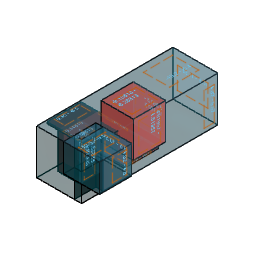
map kibo v7 (Autodesk Fusion 360 design; units mm, degrees)
Autodesk Fusion 360 part; units mm, degrees
sketch "Sketch1" plane through (0, 0, 0) normal (0, 0, 1) x (1, 0, 0)
  line L0 (12.5, 3.3758) -> (25, 3.3758)
  line L1 (25, 3.3758) -> (25, 41.3758)
  line L2 (25, 41.3758) -> (12.5, 41.3758)
  line L3 (12.5, 41.3758) -> (12.5, 3.3758)
  line L4 (93, 105.3758) -> (128, 105.3758)
  line L5 (128, 105.3758) -> (128, -41.5514)
  line L6 (23, 0.3758) -> (33, 0.3758)
  line L7 (33, 0.3758) -> (33, 9.3758)
  line L8 (33, 9.3758) -> (23, 9.3758)
  line L9 (23, 9.3758) -> (23, 0.3758)
  line L10 (20.327, 13.4945) -> (29.327, 13.4945)
  line L11 (29.327, 13.4945) -> (29.327, 22.4945)
  line L12 (29.327, 22.4945) -> (20.327, 22.4945)
  line L13 (20.327, 22.4945) -> (20.327, 13.4945)
  dimension "d1" = 12.5
  dimension "d2" = 38
  dimension "d4" = 102
  dimension "d5" = 103
  dimension "d12" = 10
  dimension "d13" = 9
  dimension "d15" = 10.5
  dimension "d17" = 3
  dimension "d50" = 9
  dimension "d51" = 9
  dimension "d53" = 3.673
  dimension "d54" = 13.1187
  constraint horizontal L0
  constraint vertical L1
  constraint horizontal L2
  constraint vertical L3
  constraint horizontal L4
  constraint perpendicular L4 L5
  constraint horizontal L6
  constraint vertical L7
  constraint horizontal L8
  constraint vertical L9
  constraint horizontal L10
  constraint vertical L11
  constraint horizontal L12
  constraint vertical L13
  measures "d1" distance of L1.end L2.end
  measures "d2" distance of L0.end L1.end
  measures "d4" distance of L0 L4
  measures "d5" distance of L1 L5
  measures "d12" distance of L6.start L6.end
  measures "d13" distance of L6.end L7.end
  measures "d15" distance of L3 L9
  measures "d17" distance of L0 L6
  measures "d50" distance of L10.start L12.end
  measures "d51" distance of L10.start L10.end
  measures "d53" distance of L7 L11
  measures "d54" distance of L6 L10
extrude "Extrude20" add sketch "Sketch1" against normal blind 48.1957 contours L1 L10 L11 L12 | L1 L10 L12 L13 makes body 1
extrude "Extrude17" add sketch "Sketch1" against normal blind 48 separate body contours L0 L1 L8 L9 makes body 2
extrude "Extrude15" add sketch "Sketch1" against normal blind 48 separate body contours L0 L1 L6 L7 L8 L9 makes body 3
extrude "Extrude12" add sketch "Sketch1" against normal blind 55.7 separate body contours L0 L1 L8 L9 makes body 4
extrude "Extrude5" add sketch "Sketch1" along normal blind 48 separate body contours L0 L1 L8 L9 makes body 5
extrude "Extrude4" add sketch "Sketch1" along normal blind 48 separate body contours L0 L1 L6 L7 L8 L9 makes body 6
extrude "Extrude2" add sketch "Sketch1" along normal blind 55.7 separate body contours L0 L1 L2 L3 L8 L9 L10 L12 L13 | L0 L1 L8 L9 | L1 L10 L12 L13 makes body 7
extrude "Extrude1" add sketch "Sketch1" along normal blind 12.5 separate body contours L0 L1 L2 L3 L8 L9 L10 L12 L13 | L0 L1 L8 L9 | L1 L10 L12 L13 makes body 8
extrude "Extrude3" cut sketch "Sketch1" along normal blind 43.2 contours L0 L1 L2 L3 L8 L9 L10 L12 L13 | L0 L1 L8 L9 | L1 L10 L12 L13 bodies 7 8
extrude "Extrude6" cut sketch "Sketch1" along normal blind 40.2 contours L0 L1 L6 L7 L8 L9 bodies 6
extrude "Extrude7" cut sketch "Sketch1" along normal blind 40.2 contours L0 L1 L8 L9 bodies 5
extrude "Extrude8" cut 1 faces at (20.8333, 16.0424, 55.7) along direction (0, 0, -1) blind 15 on bodies 7 bodies 5 7
extrude "Extrude9" cut 1 faces at (30.3333, 4.3758, 48) along direction (0, 0, -1) blind 10 on bodies 6 bodies 6
extrude "Extrude10" cut 1 faces at (23.6667, 7.3758, 40.7) along direction (0, 0, -1) blind 1 on bodies 5 bodies 5
extrude "Extrude11" add sketch "Sketch1" against normal blind 55.7 contours L0 L1 L2 L3 L8 L9 L10 L12 L13 | L1 L10 L12 L13 bodies 5 6 7 8
extrude "Extrude13" cut sketch "Sketch1" against normal blind 43.2 contours L0 L1 L2 L3 L8 L9 L10 L12 L13 | L1 L10 L12 L13 bodies 5
extrude "Extrude14" cut sketch "Sketch1" against normal blind 43.2 contours L0 L1 L8 L9 bodies 4
extrude "Extrude16" cut sketch "Sketch1" against normal blind 48 contours L0 L1 L8 L9 bodies 4
extrude "Extrude18" cut sketch "Sketch1" against normal blind 40.2 contours L0 L1 L6 L7 L8 L9 bodies 3
extrude "Extrude19" cut sketch "Sketch1" against normal blind 40.2 contours L0 L1 L8 L9 bodies 2
extrude "Extrude21" cut sketch "Sketch1" against normal blind 38.1957 contours L1 L10 L11 L12 | L1 L10 L12 L13 bodies 1
sketch "Sketch3" plane through (25, 0, 0) normal (1, 0, 0) x (0, 1, 0)
  line L0 (41.3758, -43.2) -> (9.3758, -43.2)
  line L1 (9.3758, -43.2) -> (9.3758, -55.7)
  line L2 (9.3758, -55.7) -> (41.3758, -55.7)
  line L3 (41.3758, -55.7) -> (41.3758, -43.2)
  line L4 (10.8758, -48.2063) -> (20.3758, -48.2063)
  line L5 (20.3758, -48.2063) -> (20.3758, -48.7063)
  line L6 (20.3758, -48.7063) -> (10.8758, -48.7063)
  line L7 (10.8758, -48.7063) -> (10.8758, -48.2063)
  dimension "d68" = 0.5
  dimension "d69" = 9.5
  dimension "d70" = 30.5
  dimension "d71" = 5.0063
  constraint horizontal L4
  constraint vertical L5
  constraint horizontal L6
  constraint vertical L7
  measures "d68" distance of L4.start L6.end
  measures "d69" distance of L5.end L6.end
  measures "d70" distance of L3 L7
  measures "d71" distance of L0 L4
extrude "Extrude23" add sketch "Sketch3" against normal blind 54 separate body contours L4 L5 L6 L7 makes body 9
extrude "Extrude22" add sketch "Sketch3" along normal blind 4.415 contours L4 L5 L6 L7 bodies 5
extrude "Extrude24" add sketch "Sketch3" along normal blind 9 contours L4 L5 L6 L7 bodies 9
extrude "Extrude25" cut 1 faces at (34, 17.2091, -48.5396) along direction (-1, 0, 0) blind 9 on bodies 9 bodies 9
extrude "Extrude26" add sketch "Sketch3" along normal blind 4.415 contours L4 L5 L6 L7 bodies 9
extrude "Extrude27" cut 1 faces at (-29, 17.2091, -48.5396) along direction (1, 0, 0) blind 35 on bodies 9 bodies 9
extrude "Extrude28" cut 1 faces at (6, 17.2091, -48.5396) along direction (1, 0, 0) blind 1.915 on bodies 9 bodies 9
sketch "Sketch4" plane through (0, 41.3758, 0) normal (0, 1, 0) x (-1, 0, 0)
  line L0 (-12.5, -43.2) -> (-25, -43.2)
  line L1 (-25, -43.2) -> (-25, -55.7)
  line L2 (-25, -55.7) -> (-12.5, -55.7)
  line L3 (-12.5, -55.7) -> (-12.5, -43.2)
  line L4 (-16.933, -48.7385) -> (-10.933, -48.7385)
  line L5 (-10.933, -48.7385) -> (-10.933, -58.7385)
  line L6 (-10.933, -58.7385) -> (-16.933, -58.7385)
  line L7 (-16.933, -58.7385) -> (-16.933, -48.7385)
  line L8 (-25, -55.7) -> (-25, -43.2)
  dimension "d86" = 10
  dimension "d87" = 5.5385
  dimension "d88" = 12.5
  dimension "d89" = 8.067
  constraint horizontal L4
  constraint vertical L5
  constraint horizontal L6
  constraint vertical L7
  measures "d86" distance of L4 L6
  measures "d87" distance of L0 L4
  measures "d88" distance of L0 L2
  measures "d89" distance of L7 L8
extrude "Extrude29" add sketch "Sketch4" against normal blind 30.4819 separate body contours L2 L3 L4 L5 L6 L7 | L2 L3 L4 L7 makes body 10
extrude "Extrude30" cut 1 faces at (13.4553, 41.3758, -54.3923) along direction (0, -1, 0) blind 24.9819 on bodies 10 bodies 10
sketch "Sketch5" plane through (0, 41.3758, 0) normal (0, 1, 0) x (-1, 0, 0)
  line L0 (-12.5, -43.2) -> (-25, -43.2)
  line L1 (-25, -43.2) -> (-25, -55.7)
  line L2 (-25, -55.7) -> (-12.5, -55.7)
  line L3 (-12.5, -55.7) -> (-12.5, -43.2)
  line L4 (-22.2172, -53.0788) -> (-13.731, -53.0067) construction
  line L5 (-13.731, -53.0067) -> (-13.7828, -46.9212) construction
  line L6 (-13.7828, -46.9212) -> (-22.269, -46.9933) construction
  line L7 (-22.269, -46.9933) -> (-22.2172, -53.0788) construction
  dimension "d94" = 1
sketch "Sketch6" plane through (0, 0, -43.2) normal (0, 0, 1) x (-1, 0, 0)
  line L0 (-25, -9.3758) -> (-25, -41.3758)
  line L1 (-25, -41.3758) -> (-12.5, -41.3758)
  line L2 (-12.5, -41.3758) -> (-12.5, -3.3758)
  line L3 (-12.5, -3.3758) -> (-23, -3.3758)
  line L4 (-23, -3.3758) -> (-23, -9.3758)
  line L5 (-23, -9.3758) -> (-25, -9.3758)
  line L6 (-14.3489, -39.3828) -> (-14.4534, -31.2092) construction
  line L7 (-14.4534, -31.2092) -> (-21.6785, -31.3016) construction
  line L8 (-21.6785, -31.3016) -> (-21.574, -39.4751) construction
  line L9 (-21.574, -39.4751) -> (-14.3489, -39.3828) construction
  dimension "d95" = 1
sketch "Sketch7" plane through (25, 0, 0) normal (1, 0, 0) x (0, 1, 0)
  line L0 (10.8758, -48.7063) -> (10.8758, -48.2063)
  line L1 (10.8758, -48.2063) -> (20.3758, -48.2063)
  line L2 (20.3758, -48.2063) -> (20.3758, -48.7063)
  line L3 (20.3758, -48.7063) -> (10.8758, -48.7063)
  line L4 (41.3758, -43.2) -> (9.3758, -43.2)
  line L5 (9.3758, -43.2) -> (9.3758, -55.7)
  line L6 (9.3758, -55.7) -> (41.3758, -55.7)
  line L7 (41.3758, -55.7) -> (41.3758, -43.2)
  line L8 (37.5325, -45.4907) -> (37.5706, -54.6349) construction
  line L9 (37.5706, -54.6349) -> (40.398, -54.6231) construction
  line L10 (40.398, -54.6231) -> (40.3599, -45.4789) construction
  line L11 (40.3599, -45.4789) -> (37.5325, -45.4907) construction
  dimension "d96" = 1
sketch "Sketch8" plane through (0, 0, -38.1957) normal (0, 0, 1) x (-1, 0, 0)
  line L0 (-20.327, -22.4945) -> (-20.327, -13.4945)
  line L1 (-20.327, -13.4945) -> (-29.327, -13.4945)
  line L2 (-29.327, -13.4945) -> (-29.327, -22.4945)
  line L3 (-29.327, -22.4945) -> (-20.327, -22.4945)
  line L4 (-27.9693, -14.4737) -> (-28.0105, -21.4912) construction
  line L5 (-28.0105, -21.4912) -> (-22.0307, -21.5263) construction
  line L6 (-22.0307, -21.5263) -> (-21.9895, -14.5088) construction
  line L7 (-21.9895, -14.5088) -> (-27.9693, -14.4737) construction
  dimension "d97" = 1
sketch "Sketch9" plane through (0, 22.4945, 0) normal (0, 1, 0) x (-1, 0, 0)
  line L0 (-20.327, -38.1957) -> (-29.327, -38.1957)
  line L1 (-29.327, -38.1957) -> (-29.327, -48.1957)
  line L2 (-29.327, -48.1957) -> (-20.327, -48.1957)
  line L3 (-20.327, -48.1957) -> (-20.327, -38.1957)
sketch "Sketch10" plane through (0, 22.4945, 0) normal (0, 1, 0) x (-1, 0, 0)
  line L0 (-20.327, -38.1957) -> (-29.327, -38.1957)
  line L1 (-29.327, -38.1957) -> (-29.327, -48.1957)
  line L2 (-29.327, -48.1957) -> (-20.327, -48.1957)
  line L3 (-20.327, -48.1957) -> (-20.327, -38.1957)
  line L4 (-28.3912, -46.8098) -> (-20.9328, -46.7616) construction
  line L5 (-20.9328, -46.7616) -> (-20.9767, -39.9699) construction
  line L6 (-20.9767, -39.9699) -> (-28.4351, -40.0181) construction
  line L7 (-28.4351, -40.0181) -> (-28.3912, -46.8098) construction
  dimension "d98" = 1
sketch "Sketch11" plane through (29.327, 0, 0) normal (1, 0, 0) x (0, 1, 0)
  line L0 (22.4945, -38.1957) -> (13.4945, -38.1957)
  line L1 (13.4945, -38.1957) -> (13.4945, -48.1957)
  line L2 (13.4945, -48.1957) -> (22.4945, -48.1957)
  line L3 (22.4945, -48.1957) -> (22.4945, -38.1957)
  line L4 (15, -39.3888) -> (15, -47.3888) construction
  line L5 (15, -47.3888) -> (21, -47.3888) construction
  line L6 (21, -47.3888) -> (21, -39.3888) construction
  line L7 (21, -39.3888) -> (15, -39.3888) construction
  dimension "d99" = 1
sketch "Sketch12" plane through (0, 16.3939, 0) normal (0, 1, 0) x (-1, 0, 0)
  line L0 (-16.933, -58.7385) -> (-10.933, -58.7385)
  line L1 (-10.933, -58.7385) -> (-10.933, -48.7385)
  line L2 (-10.933, -48.7385) -> (-16.933, -48.7385)
  line L3 (-16.933, -48.7385) -> (-16.933, -58.7385)
  line L4 (-15.9994, -55.0006) -> (-12.0006, -55.0007) construction
  line L5 (-12.0006, -55.0007) -> (-12.0006, -50.9994) construction
  line L6 (-12.0006, -50.9994) -> (-15.9994, -50.9993) construction
  line L7 (-15.9994, -50.9993) -> (-15.9994, -55.0006) construction
  dimension "d100" = 1
sketch "Sketch13" plane through (16.933, 0, 0) normal (1, 0, 0) x (0, 1, 0)
  line L0 (16.3939, -58.7385) -> (16.3939, -48.7385)
  line L1 (16.3939, -48.7385) -> (10.8939, -48.7385)
  line L2 (10.8939, -48.7385) -> (10.8939, -58.7385)
  line L3 (10.8939, -58.7385) -> (16.3939, -58.7385)
  line L4 (12.1736, -50.3905) -> (12.1736, -58.3905) construction
  line L5 (12.1736, -58.3905) -> (15.1736, -58.3905) construction
  line L6 (15.1736, -58.3905) -> (15.1736, -50.3905) construction
  line L7 (15.1736, -50.3905) -> (12.1736, -50.3905) construction
  dimension "d101" = 1
sketch "Sketch14" plane through (0, 0, -48.7385) normal (0, 0, 1) x (-1, 0, 0)
  line L0 (-16.933, -16.3939) -> (-10.933, -16.3939)
  line L1 (-10.933, -16.3939) -> (-10.933, -10.8939)
  line L2 (-10.933, -10.8939) -> (-16.933, -10.8939)
  line L3 (-16.933, -10.8939) -> (-16.933, -16.3939)
  line L4 (-16.1399, -11.247) -> (-16.1685, -15.8024) construction
  line L5 (-16.1685, -15.8024) -> (-11.9578, -15.8289) construction
  line L6 (-11.9578, -15.8289) -> (-11.9292, -11.2735) construction
  line L7 (-11.9292, -11.2735) -> (-16.1399, -11.247) construction
  dimension "d102" = 0.9
sketch "Sketch15" plane through (0, 20.3758, 0) normal (0, 1, 0) x (-1, 0, 0)
  line L0 (-7.915, -48.7063) -> (-7.915, -48.2063)
  line L1 (-7.915, -48.2063) -> (-29.415, -48.2063)
  line L2 (-29.415, -48.2063) -> (-29.415, -48.7063)
  line L3 (-29.415, -48.7063) -> (-7.915, -48.7063)
  line L4 (-20.81, -48.7063) -> (-12.8433, -48.7063) construction
  line L5 (-12.8433, -48.7063) -> (-12.8433, -48.2063) construction
  line L6 (-12.8433, -48.2063) -> (-20.81, -48.2063) construction
  line L7 (-20.81, -48.2063) -> (-20.81, -48.7063) construction
  dimension "d103" = 0.4
  constraint coincident L3
  constraint coincident L1
sketch "Sketch16" plane through (0, 0, -48.2063) normal (0, 0, 1) x (-1, 0, 0)
  line L0 (-7.915, -20.3758) -> (-7.915, -10.8758)
  line L1 (-7.915, -10.8758) -> (-29.415, -10.8758)
  line L2 (-29.415, -10.8758) -> (-29.415, -20.3758)
  line L3 (-29.415, -20.3758) -> (-7.915, -20.3758)
  line L4 (-11.34, -12.425) -> (-11.34, -19.425) construction
  line L5 (-11.34, -19.425) -> (-8.34, -19.425) construction
  line L6 (-8.34, -19.425) -> (-8.34, -12.425) construction
  line L7 (-8.34, -12.425) -> (-11.34, -12.425) construction
  dimension "d104" = 0.9
sketch "Sketch17" plane through (29.415, 0, 0) normal (1, 0, 0) x (0, 1, 0)
  line L0 (10.8758, -48.7063) -> (20.3758, -48.7063)
  line L1 (20.3758, -48.7063) -> (20.3758, -48.2063)
  line L2 (20.3758, -48.2063) -> (10.8758, -48.2063)
  line L3 (10.8758, -48.2063) -> (10.8758, -48.7063)
  line L4 (13.1314, -48.7063) -> (18.276, -48.7063) construction
  line L5 (18.276, -48.7063) -> (18.276, -48.2063) construction
  line L6 (18.276, -48.2063) -> (13.1314, -48.2063) construction
  line L7 (13.1314, -48.2063) -> (13.1314, -48.7063) construction
  dimension "d105" = 0.4
  constraint coincident L0
  constraint coincident L2
sketch "Sketch18" plane through (0, 9.3758, 0) normal (0, 1, 0) x (-1, 0, 0)
  line L0 (-25, -40.2) -> (-33, -40.2)
  line L1 (-33, -40.2) -> (-33, -48)
  line L2 (-33, -48) -> (-25, -48)
  line L3 (-25, -48) -> (-25, -40.2)
  line L4 (-31.5434, -45.7991) -> (-25.5434, -45.7991) construction
  line L5 (-25.5434, -45.7991) -> (-25.5434, -41.7991) construction
  line L6 (-25.5434, -41.7991) -> (-31.5434, -41.7991) construction
  line L7 (-31.5434, -41.7991) -> (-31.5434, -45.7991) construction
  dimension "d106" = 1
sketch "Sketch19" plane through (0, 0, -40.2) normal (0, 0, 1) x (-1, 0, 0)
  line L0 (-23, -3.3758) -> (-23, -0.3758)
  line L1 (-23, -0.3758) -> (-33, -0.3758)
  line L2 (-33, -0.3758) -> (-33, -9.3758)
  line L3 (-33, -9.3758) -> (-25, -9.3758)
  line L4 (-25, -9.3758) -> (-25, -3.3758)
  line L5 (-25, -3.3758) -> (-23, -3.3758)
  line L6 (-30.3839, -0.9918) -> (-30.3839, -8.4119) construction
  line L7 (-30.3839, -8.4119) -> (-26.5788, -8.4119) construction
  line L8 (-26.5788, -8.4119) -> (-26.5788, -0.9918) construction
  line L9 (-26.5788, -0.9918) -> (-30.3839, -0.9918) construction
  dimension "d107" = 1
sketch "Sketch20" plane through (33, 0, 0) normal (1, 0, 0) x (0, 1, 0)
  line L0 (9.3758, -40.2) -> (0.3758, -40.2)
  line L1 (0.3758, -40.2) -> (0.3758, -48)
  line L2 (0.3758, -48) -> (9.3758, -48)
  line L3 (9.3758, -48) -> (9.3758, -40.2)
  line L4 (4, -41) -> (4, -47) construction
  line L5 (4, -47) -> (8, -47) construction
  line L6 (8, -47) -> (8, -41) construction
  line L7 (8, -41) -> (4, -41) construction
  dimension "d108" = 1
extrude "Extrude31" cut 1 faces at (29.415, 17.2091, -48.5396) along direction (-1, 0, 0) blind 4.5 on bodies 5 bodies 5
extrude "Extrude32" add 1 faces at (24.915, 17.2091, -48.5396) along direction (1, 0, 0) blind 0.1 on bodies 5 bodies 5
